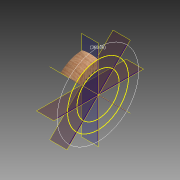
# Autodesk Inventor part: bigWheelWedge01
Saved by Autodesk Inventor 2013 (Build 170138000, 138)
## iProperties
Created: 2013-01-08
Part Number: bigWheelWedge01
Material: Wood (Maple)
Document SubType Name: Modeling
Designer: Nano
Density: 0.57 g/cm^3
Mass: 2208.67 g
Surface Area: 1950.19 cm^2
Volume: 3874.85 cm^3
Author: Nano
Autodesk Inventor part; units mm, degrees
note: some values were not read from the file. Chosen so that the rebuilt part matches the saved one: copy form of "Circular Pattern2".
ref_plane "YZ Plane" through (0, 0, 0) normal (1, 0, 0) x (0, 1, 0)
ref_plane "XZ Plane" through (0, 0, 0) normal (0, 1, 0) x (-1, 0, 0)
sketch "Sketch1" plane through (0, 0, 0) normal (0, 0, 1) x (1, 0, 0)
  circle A0 centre (0, 0) radius 139.7
  line L0 (0, 139.7) -> (234.2216, 139.7) construction
  line L1 (-34.925, 185.7375) -> (34.925, 185.7375) construction
  line L2 (34.925, 185.7375) -> (34.925, 93.6625)
  line L3 (34.925, 93.6625) -> (-34.925, 93.6625)
  line L4 (-34.925, 93.6625) -> (-34.925, 185.7375)
  line L5 (-34.925, 185.7375) -> (34.925, 93.6625) construction
  line L6 (34.925, 185.7375) -> (-34.925, 93.6625) construction
  line L7 (0, 0) -> (253.8576, 0) construction
  point P0 (-34.925, 135.2639)
  point P1 (34.925, 135.2639)
  dimension "d6" = 279.4
  dimension "d7" = 69.85
  dimension "d8" = 92.075
  dimension "d9" = 93.6625
  constraints: 16 end point, 3 point on circle, 2 horizontal, 2 midpoint, 2 parallel, 2 perpendicular, 2 point on line, 1 centre point, 1 tangent, 1 other
  measures "d6" diameter of A0
  measures "d7" distance of L2.end L3.end
  measures "d8" distance of L1.end L2.end
  measures "d9" distance from line of L7.start L3
revolve "Revolution2" add sketch "Sketch1" angle 360 about axis through (0, 0, 0) along (1, 0, 0) picked at (2.3523, 108.9489) contours L2 L3 L4 A0
sketch "Sketch4" plane through (-34.925, 0, 0) normal (-1, 0, 0) x (0, 0, 1)
  circle A0 centre (0, 0) radius 93.6625 projected
  circle A1 centre (0, 0) radius 117.475
  dimension "d24" = 234.95
  constraints: 1 centre point, 1 coincident
  measures "d24" diameter of A1
extrude "Extrusion3" cut sketch "Sketch4" against normal blind 12.7
sketch "Sketch5" plane through (34.925, 0, 0) normal (1, 0, 0) x (0, 0, -1)
  circle A0 centre (0, 0) radius 93.6625 projected
  circle A1 centre (0, 0) radius 135.2639 projected
  line L0 (0, 0) -> (0, 180.6754)
  line L1 (0, 0) -> (-127.7568, 127.7568)
  line L2 (0, 0) -> (-180.6754, 0)
  line L3 (0, 0) -> (-127.7568, -127.7568)
  line L4 (0, 0) -> (0, -180.6754)
  line L5 (0, 0) -> (127.7568, -127.7568)
  line L6 (0, 0) -> (180.6754, 0)
  line L7 (0, 0) -> (127.7568, 127.7568)
  dimension "d29" = 360
  constraints: 16 end point, 1 vertical, 25 other
ref_plane "Work Plane1" through (34.925, 0, 0) normal (0, 0, 1) x (0, 1, 0)
pattern_circular "Circular Pattern1" count 8 over 360 about axis through (0, 0, 0) along (1, 0, 0)
split "Split1" plane through (34.925, 0, 0) removes the side toward (0, 0, -1)
split "Split2" plane through (34.925, 0, 0) removes the side toward (0, -0.7071068, 0.7071068)
sketch "Sketch6" plane through (-22.225, 0, 0) normal (-1, 0, 0) x (0, 0, 1)
  arc A0 (66.2294, 66.2294) -> (0, 93.6625) centre (0, 0) ccw projected
  line L0 (0, 0) -> (75.2096, 181.5721) construction
  line L1 (0, 0) -> (196.5323, 0) construction
  line L2 (32.8892, 87.6982) -> (38.7558, 85.2681)
  line L3 (38.7558, 85.2681) -> (41.1858, 91.1348)
  line L4 (41.1858, 91.1348) -> (35.3192, 93.5648)
  line L5 (35.3192, 93.5648) -> (32.8892, 87.6982)
  line L6 (38.2525, 92.3498) -> (35.8225, 86.4831)
  dimension "d37" = 67.5
  dimension "d46" = 6.35
  dimension "d48" = 6.35
  constraints: 14 end point, 2 midpoint, 2 parallel, 1 collinear, 1 equal length, 1 horizontal, 1 perpendicular, 1 point on circle
  measures "d37" angle of L1 L0
  measures "d46" distance of L3.end L4.end
  measures "d48" distance of L2.end L3.end
extrude "Extrusion4" cut sketch "Sketch6" against normal up to next
pattern_circular "Circular Pattern2" count 40 over 360 about axis through (0, 0, 0) along (1, 0, 0) of "Extrusion4" geometry pattern yes
ref_plane "Work Plane2" through (34.925, 0, 0) normal (0, -0.7071068, 0.7071068) x (0, 0.7071068, 0.7071068)
ref_plane "Work Plane3" through (34.925, 0, 0) normal (0, -1, 0) x (0, 0, 1)
ref_plane "Work Plane4" through (34.925, 0, 0) normal (0, -0.7071068, -0.7071068) x (0, -0.7071068, 0.7071068)
ref_plane "Work Plane5" through (34.925, 0, 0) normal (0, 0, -1) x (0, -1, 0)
ref_plane "Work Plane6" through (34.925, 0, 0) normal (0, 0.7071068, -0.7071068) x (0, -0.7071068, -0.7071068)
ref_plane "Work Plane7" through (34.925, 0, 0) normal (0, 1, 0) x (0, 0, -1)
ref_plane "Work Plane8" through (34.925, 0, 0) normal (0, 0.7071068, 0.7071068) x (0, 0.7071068, -0.7071068)
body "Solid2"
